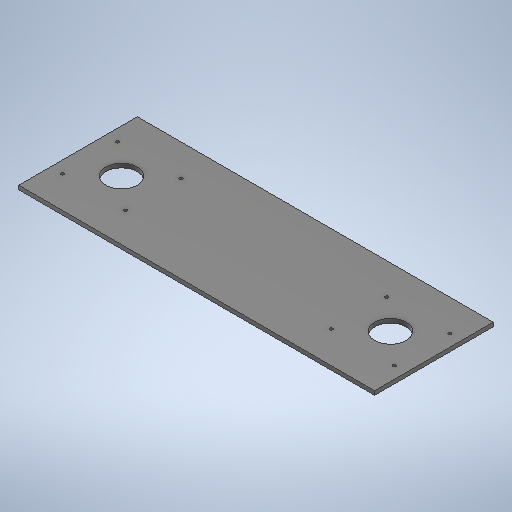
# Autodesk Inventor part: acrylic_back
Saved by Autodesk Inventor 2026.2 (Build 302298010, 298A)
## iProperties
Created: 2026-05-13
Part Number: acrylic_back
Material: ABS Plastic
Document SubType Name: Modeling
Designer: chris
Density: 1.06 g/cm^3
Appearance: Smooth - White
Author: chris
Autodesk Inventor part; units mm, degrees
ref_plane "YZ Plane" through (0, 0, 0) normal (1, 0, 0) x (0, 1, 0)
ref_plane "XZ Plane" through (0, 0, 0) normal (0, 1, 0) x (-1, 0, 0)
ref_plane "XY Plane" through (0, 0, 0) normal (0, 0, 1) x (1, 0, 0)
sketch "Sketch1" plane through (0, 0, 0) normal (0, 1, 0) x (-1, 0, 0)
  line L0 (225, 75) -> (-225, 75)
  line L1 (-225, 75) -> (-225, -75)
  line L2 (-225, -75) -> (225, -75)
  line L3 (225, -75) -> (225, 75)
  line L4 (225, 75) -> (-225, -75) construction
  line L5 (-225, 75) -> (225, -75) construction
  point P0 (0, 0)
  dimension "d0" = 450
  dimension "d1" = 150
  constraints: 12 end point, 2 midpoint, 2 parallel, 1 horizontal, 1 perpendicular
  measures "d0" distance of L2.end L1.end
  measures "d1" distance of L1.end L0.end
extrude "Extrusion1" add sketch "Sketch1" along normal blind 5
sketch "Sketch2" plane through (0, 5, 0) normal (0, 1, 0) x (1, 0, 0)
  circle A0 centre (-210, -35) radius 2.05 projected
  circle A1 centre (-130, 35) radius 2.05 projected
  circle A2 centre (-130, -35) radius 2.05 projected
  circle A3 centre (-210, 35) radius 2.05 projected
  arc A4 (-190.5, 40) -> (-194.5, 44.899) centre (-195.5, 40) ccw projected
  line L0 (-190.5, 40) -> (-190.5, -20) projected
  line L1 (-190.5, -20) -> (-149.5, -20) projected
  line L2 (-149.5, -20) -> (-149.5, 57) projected
  line L3 (-180, 57) -> (-180, 75) projected
  line L4 (-180, 75) -> (-120, 75) projected
  line L5 (-120, 75) -> (-120, -75) projected
  line L6 (-120, -75) -> (-220, -75) projected
  line L7 (-220, -75) -> (-220, 75) projected
  line L8 (-220, 75) -> (-198.5, 75) projected
  line L9 (-198.5, 75) -> (-198.5, 49.798) projected
  arc A5 (-198.5, 49.798) -> (-194.5, 44.899) centre (-193.5, 49.798) ccw projected
  circle A6 centre (-210, 35) radius 2
  circle A7 centre (-210, -35) radius 2
  circle A8 centre (-130, -35) radius 2
  circle A9 centre (-130, 35) radius 2
  line L10 (-149.5, 57) -> (-180, 57) projected
  point P0 (0, 0)
  dimension "d4" = 4
  dimension "d5" = 4
  dimension "d6" = 4
  dimension "d7" = 4
  constraints: 4 centre point, 4 coincident
  measures "d4" diameter of A6
  measures "d5" diameter of A7
  measures "d6" diameter of A8
  measures "d7" diameter of A9
extrude "Extrusion2" cut sketch "Sketch2" against normal blind 5 contours A6 | A7 | A8 | A9
mirror "Mirror1" about plane through (0, 0, 0) normal (1, 0, 0) of "Extrusion2"
sketch "Sketch4" plane through (0, 0, 0) normal (0, -1, 0) x (1, 0, 0)
  line L0 (62, 45) -> (62, 5) projected
  circle A0 centre (210, -35) radius 2 projected
  circle A1 centre (130, -35) radius 2 projected
  circle A2 centre (210, 35) radius 2 projected
  circle A3 centre (130, 35) radius 2 projected
  circle A4 centre (-130, 35) radius 2 projected
  circle A5 centre (-210, 35) radius 2 projected
  circle A6 centre (-130, -35) radius 2 projected
  circle A7 centre (-210, -35) radius 2 projected
  line L1 (225, 75) -> (225, -75) projected
  line L2 (-225, 75) -> (225, 75) projected
  line L3 (-225, -75) -> (-225, 75) projected
  line L4 (225, -75) -> (-225, -75) projected
  circle A8 centre (-170, 0) radius 20
  circle A9 centre (170, 0) radius 20
  point P0 (0, 0)
  dimension "d16" = 40
  dimension "d17" = 40
  constraints: 2 centre point
  measures "d16" diameter of A8
  measures "d17" diameter of A9
extrude "Extrusion4" cut sketch "Sketch4" against normal blind 5 contours A8 | A9
body "Solid1"
